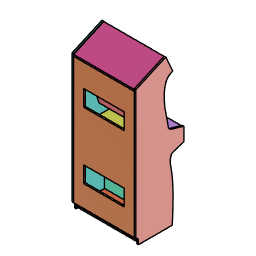
arcade_design (Autodesk Fusion 360 design; units mm, degrees)
Autodesk Fusion 360 part; units mm, degrees
sketch "Side Panels" plane through (0, 0, 0) normal (1, 0, 0) x (0, 1, 0)
  line L0 (31.75, 0) -> (457.2, 0)
  line L1 (452.7885, 785.6533) -> (609.6, 837.3077)
  line L2 (609.6, 837.3077) -> (609.6, 1002.4077)
  line L3 (609.6, 1002.4077) -> (444.4309, 1049.7691)
  line L4 (408.5002, 1089.2565) -> (363.7179, 1328.5488)
  line L5 (463.7201, 1671.9295) -> (375.9057, 1869.164)
  line L6 (0, 82.55) -> (0, 1701.8)
  line L7 (375.9057, 1869.164) -> (0, 1701.8)
  line L8 (0, 0) -> (31.75, 0)
  line L9 (31.75, 0) -> (31.75, 50.8)
  arc A0 (31.75, 50.8) -> (0, 82.55) centre (0, 50.8) ccw
  spline S0 degree 5 poles (463.7201, 1671.9295) (458.0026, 1670.3002) (446.9286, 1666.533) (431.4003, 1659.3565) (412.8977, 1646.6853) (393.6414, 1625.3901) (378.472, 1598.336) (367.4495, 1565.4385) (360.3055, 1527.0756) (356.6509, 1483.7958) (356.0894, 1436.1574) (357.8593, 1394.9197) (360.3453, 1362.3589) (362.5093, 1339.9378) (363.7179, 1328.5488) knots 0 0 0 0 0 0 0.1 0.2 0.3 0.4 0.5 0.6 0.7 0.8 0.9 1 1 1 1 1 1
  spline S1 degree 5 poles (452.7885, 785.6533) (450.1173, 780.6819) (445.2009, 770.7662) (439.1046, 755.9734) (433.5518, 736.4131) (430.8508, 711.9873) (432.0376, 686.8334) (436.2286, 659.4045) (442.2622, 627.782) (448.9298, 590.0685) (455.2454, 544.8887) (460.5567, 491.5686) (464.4393, 429.8652) (466.6536, 359.8453) (467.0872, 281.7419) (465.7134, 195.857) (463.1837, 121.152) (460.4968, 61.8426) (458.357, 20.8555) (457.2, 0) knots 0 0 0 0 0 0 0.066667 0.133333 0.2 0.266667 0.333333 0.4 0.466667 0.533333 0.6 0.666667 0.733333 0.8 0.866667 0.933333 1 1 1 1 1 1
  arc A1 (408.5002, 1089.2565) -> (444.4309, 1049.7691) centre (458.4333, 1098.6012) ccw
  point P0 (414.2716, 1058.4172)
  point P1 (31.75, 82.55)
  point P2 (381, 1600.2)
  point P3 (431.8, 711.2)
  point P4 (446.1027, 605.186)
  dimension "d1" = 457.2
  dimension "d3" = 165.1
  dimension "d5" = 165.1
  dimension "d6" = 203.2
  dimension "d7" = 106
  dimension "d8" = 10.6
  dimension "d9" = 1701.8
  dimension "d10" = 411.48
  dimension "d11" = 114
  dimension "d12" = 215.9
  dimension "d13" = 31.75
  dimension "d14" = 82.55
  dimension "d15" = 31.75
  dimension "d18" = 50.8
  dimension "d37" = 609.6
  constraint coincident L8.start origin
  constraint horizontal L0
  constraint vertical L2
  constraint perpendicular L0 L6
  constraint coincident L6 L7.end
  constraint perpendicular L5 L7
  constraint perpendicular L6 L8
  constraint perpendicular L0 L9
  constraint coincident P1 L9
  constraint tangent L9 A0
  constraint coincident P0 L3
  constraint coincident P0 L4
  constraint tangent L3 A1
  constraint tangent L4 A1
  measures "d1" distance of L8.start L0.end
  measures "d3" distance of L1.start L1.end
  measures "d5" distance of L1.end L2.end
  measures "d6" distance of L2.end P0
  measures "d7" angle of L2 L3
  measures "d8" angle of L4 L6
  measures "d9" distance of L8.start L6.end
  measures "d10" distance of L5.end L6.end
  measures "d11" angle of L6 L7
  measures "d12" distance of L5.start L5.end
  measures "d13" distance of L8.start L0.start
  measures "d14" distance of L0.start P1
  measures "d15" radius of A0
  measures "d18" radius of A1
  measures "d37" distance of L2 L6
extrude "Extrude1" add sketch "Side Panels" along normal blind 19.05 makes body 1 in component "Right Panel"
extrude "Extrude1'" add sketch "Side Panels" along normal blind 19.05 separate body makes body 2 in component "Left Panel"
sketch "Main Panels" plane through (19.05, 0, 0) normal (1, 0, 0) x (0, 1, 0)
  line L0 (463.7201, 1671.9295) -> (375.9057, 1869.164)
  line L1 (375.9057, 1869.164) -> (0, 1701.8)
  line L2 (0, 1701.8) -> (0, 82.55)
  arc A0 (31.75, 50.8) -> (0, 82.55) centre (0, 50.8) ccw
  line L3 (31.75, 50.8) -> (31.75, 0)
  line L4 (31.75, 0) -> (457.2, 0)
  spline S0 degree 5 poles (457.2, 0) (458.357, 20.8555) (460.4968, 61.8426) (463.1837, 121.152) (465.7134, 195.857) (467.0872, 281.7419) (466.6536, 359.8453) (464.4393, 429.8652) (460.5567, 491.5686) (455.2454, 544.8887) (448.9298, 590.0685) (442.2622, 627.782) (436.2286, 659.4045) (432.0376, 686.8334) (430.8508, 711.9873) (433.5518, 736.4131) (439.1046, 755.9734) (445.2009, 770.7662) (450.1173, 780.6819) (452.7885, 785.6533) knots -1 -1 -1 -1 -1 -1 -0.933333 -0.866667 -0.8 -0.733333 -0.666667 -0.6 -0.533333 -0.466667 -0.4 -0.333333 -0.266667 -0.2 -0.133333 -0.066667 0 0 0 0 0 0
  line L5 (452.7885, 785.6533) -> (609.6, 837.3077)
  line L6 (609.6, 837.3077) -> (609.6, 1002.4077)
  line L7 (609.6, 1002.4077) -> (444.4309, 1049.7691)
  arc A1 (408.5002, 1089.2565) -> (444.4309, 1049.7691) centre (458.4333, 1098.6012) ccw
  line L8 (408.5002, 1089.2565) -> (363.7179, 1328.5488)
  spline S1 degree 5 poles (363.7179, 1328.5488) (362.5093, 1339.9378) (360.3453, 1362.3589) (357.8593, 1394.9197) (356.0894, 1436.1574) (356.6509, 1483.7958) (360.3055, 1527.0756) (367.4495, 1565.4385) (378.472, 1598.336) (393.6414, 1625.3901) (412.8977, 1646.6853) (431.4003, 1659.3565) (446.9286, 1666.533) (458.0026, 1670.3002) (463.7201, 1671.9295) knots -1 -1 -1 -1 -1 -1 -0.9 -0.8 -0.7 -0.6 -0.5 -0.4 -0.3 -0.2 -0.1 0 0 0 0 0 0
  line L9 (375.9057, 1869.164) -> (383.654, 1851.761)
  line L10 (383.654, 1851.761) -> (0, 1680.9472)
  line L11 (0, 1680.9472) -> (0, 1701.8)
  line L12 (0, 1701.8) -> (375.9057, 1869.164)
  line L13 (0, 1680.9472) -> (0, 82.55)
  line L14 (0, 82.55) -> (19.05, 82.55)
  line L15 (19.05, 82.55) -> (19.05, 1689.4288)
  line L16 (463.7201, 1671.9295) -> (455.9718, 1689.3326)
  line L17 (455.9718, 1689.3326) -> (160.5069, 1557.7831)
  line L18 (166.4261, 1539.5657) -> (463.7201, 1671.9295)
  line L19 (406.3216, 0) -> (406.3216, 862.4074)
  line L20 (406.3216, 862.4074) -> (387.2716, 862.4074)
  line L21 (387.2716, 862.4074) -> (387.2716, 0)
  line L22 (565.0941, 983.0574) -> (584.1441, 983.0574)
  line L23 (584.1441, 983.0574) -> (584.1441, 881.4574)
  line L24 (584.1441, 881.4574) -> (565.0941, 881.4574)
  line L25 (565.0941, 881.4574) -> (565.0941, 983.0574)
  line L26 (565.0941, 881.4574) -> (565.0941, 862.4074)
  line L27 (565.0941, 862.4074) -> (184.0941, 862.4074)
  line L28 (184.0941, 862.4074) -> (184.0941, 881.4574)
  line L29 (184.0941, 881.4574) -> (565.0941, 881.4574)
  line L30 (598.8774, 1003.0679) -> (597.2171, 984.0904)
  line L31 (597.2171, 984.0904) -> (339.5874, 1006.63)
  line L32 (333.1923, 1026.3123) -> (598.8774, 1003.0679)
  line L33 (565.0941, 983.0574) -> (355.6, 983.0574) construction
  line L34 (333.1923, 1026.3123) -> (166.4261, 1539.5657)
  line L35 (333.1923, 1026.3123) -> (339.5874, 1006.63)
  line L36 (166.4261, 1539.5657) -> (160.5069, 1557.7831)
  line L37 (154.343, 1576.7538) -> (136.2254, 1570.867)
  line L38 (136.2254, 1570.867) -> (321.4698, 1000.7433)
  line L39 (339.5874, 1006.63) -> (321.4698, 1000.7433)
  line L40 (154.343, 1576.7538) -> (166.4261, 1539.5657)
  dimension "d19" = 19.05
  dimension "d20" = 19.05
  dimension "d21" = 19.05
  dimension "d23" = 19.05
  dimension "d27" = 19.05
  dimension "d28" = 101.6
  dimension "d29" = 19.05
  dimension "d30" = 381
  dimension "d31" = 19.05
  dimension "d32" = 266.7
  dimension "d33" = 5
  dimension "d34" = 18
  dimension "d36" = 19.05
  constraint coincident L0.end L1.start
  constraint coincident L0 L9.end
  constraint coincident L2 L10.end
  constraint perpendicular L0 L10
  constraint coincident L1.end L2.start
  constraint coincident L2.end A0.end
  constraint perpendicular L2 L14
  constraint coincident L10 L15.end
  constraint perpendicular L14 L15
  constraint coincident L0.start S1.end
  constraint parallel L0 L16
  constraint perpendicular L0 L17
  constraint perpendicular L0 L18
  constraint coincident L4 L19.start
  constraint perpendicular L4 L19
  constraint perpendicular L19 L20
  constraint coincident L4 L21.end
  constraint perpendicular L4 L21
  constraint horizontal L22
  constraint perpendicular L22 L23
  constraint perpendicular L23 L24
  constraint perpendicular L22 L25
  constraint perpendicular L24 L26
  constraint perpendicular L21 L27
  constraint perpendicular L27 L28
  constraint perpendicular L30 L31
  constraint parallel L31 L32
  constraint perpendicular L25 L33
  constraint coincident L19.end L27
  constraint parallel L34 L35
  constraint parallel L34 L36
  constraint perpendicular L36 L37
  constraint perpendicular L37 L38
  constraint perpendicular L38 L39
  constraint perpendicular L37 L40
  measures "d19" distance of L0.end L9.end
  measures "d20" distance of L2.end L14.end
  measures "d21" distance of L0.start L16.end
  measures "d23" distance of L19.end L20.end
  measures "d27" distance of L22.start L22.end
  measures "d28" distance of L22.end L23.end
  measures "d29" distance of L24.end L26.end
  measures "d30" distance of L26.end L27.end
  measures "d31" distance of L30.start L30.end
  measures "d32" distance of L30.start L32.start
  measures "d33" angle of L31 L33
  measures "d34" angle of L15 L34
  measures "d36" distance of L37.start L37.end
extrude "Extrude1''" add sketch "Main Panels" along normal blind 711.2 separate body contours L2 L10 L13 L14 L15 makes body 3 in component "Back Panel"
extrude "Extrude1'''" add sketch "Main Panels" along normal blind 711.2 separate body contours L34 L35 L36 L37 L38 L39 L40 makes body 4 in component "Screen Panel"
extrude "Extrude1''''" add sketch "Main Panels" along normal blind 711.2 separate body contours L30 L31 L32 L35 makes body 5 in component "Control Panel"
extrude "Extrude1'''''" add sketch "Main Panels" along normal blind 711.2 separate body contours L22 L23 L24 L25 makes body 6 in component "Tray Door"
extrude "Extrude1''''''" add sketch "Main Panels" along normal blind 711.2 separate body contours L20 L26 L27 L28 L29 makes body 7 in component "Tray Bottom"
extrude "Extrude1'''''''" add sketch "Main Panels" along normal blind 711.2 separate body contours L4 L19 L20 L21 L27 makes body 8 in component "Front Panel"
sketch "Keyboard Tray" plane through (19.05, 0, 0) normal (1, 0, 0) x (0, 1, 0)
  line L0 (463.7201, 1671.9295) -> (375.9057, 1869.164)
  line L1 (375.9057, 1869.164) -> (0, 1701.8)
  line L2 (0, 1701.8) -> (0, 82.55)
  arc A0 (31.75, 50.8) -> (0, 82.55) centre (0, 50.8) ccw
  line L3 (31.75, 50.8) -> (31.75, 0)
  line L4 (31.75, 0) -> (457.2, 0)
  spline S0 degree 5 poles (457.2, 0) (458.357, 20.8555) (460.4968, 61.8426) (463.1837, 121.152) (465.7134, 195.857) (467.0872, 281.7419) (466.6536, 359.8453) (464.4393, 429.8652) (460.5567, 491.5686) (455.2454, 544.8887) (448.9298, 590.0685) (442.2622, 627.782) (436.2286, 659.4045) (432.0376, 686.8334) (430.8508, 711.9873) (433.5518, 736.4131) (439.1046, 755.9734) (445.2009, 770.7662) (450.1173, 780.6819) (452.7885, 785.6533) knots -1 -1 -1 -1 -1 -1 -0.933333 -0.866667 -0.8 -0.733333 -0.666667 -0.6 -0.533333 -0.466667 -0.4 -0.333333 -0.266667 -0.2 -0.133333 -0.066667 0 0 0 0 0 0
  line L5 (452.7885, 785.6533) -> (609.6, 837.3077)
  line L6 (609.6, 837.3077) -> (609.6, 1002.4077)
  line L7 (609.6, 1002.4077) -> (444.4309, 1049.7691)
  arc A1 (408.5002, 1089.2565) -> (444.4309, 1049.7691) centre (458.4333, 1098.6012) ccw
  line L8 (408.5002, 1089.2565) -> (363.7179, 1328.5488)
  spline S1 degree 5 poles (363.7179, 1328.5488) (362.5093, 1339.9378) (360.3453, 1362.3589) (357.8593, 1394.9197) (356.0894, 1436.1574) (356.6509, 1483.7958) (360.3055, 1527.0756) (367.4495, 1565.4385) (378.472, 1598.336) (393.6414, 1625.3901) (412.8977, 1646.6853) (431.4003, 1659.3565) (446.9286, 1666.533) (458.0026, 1670.3002) (463.7201, 1671.9295) knots -1 -1 -1 -1 -1 -1 -0.9 -0.8 -0.7 -0.6 -0.5 -0.4 -0.3 -0.2 -0.1 0 0 0 0 0 0
  line L9 (267.3124, 912.0538) -> (546.7124, 912.0538)
  line L10 (546.7124, 912.0538) -> (546.7124, 893.0038)
  line L11 (546.7124, 893.0038) -> (267.3124, 893.0038)
  line L12 (267.3124, 893.0038) -> (267.3124, 912.0538)
  dimension "d54" = 279.4
  dimension "d55" = 19.05
  constraint horizontal L9
  constraint vertical L10
  constraint horizontal L11
  constraint vertical L12
  measures "d54" distance of L9.start L9.end
  measures "d55" distance of L9.start L11.end
extrude "Extrude1''''''''" add sketch "Keyboard Tray" along normal blind 711.2 separate body contours L9 L10 L11 L12 makes body 9 in component "Keyboard Tray"
sketch "Coin Door" plane through (0, 406.3216, 0) normal (0, 1, 0) x (-1, 0, 0)
  line L0 (-19.05, 0) -> (-19.05, 862.4074)
  line L1 (-19.05, 862.4074) -> (-730.25, 862.4074)
  line L2 (-730.25, 862.4074) -> (-730.25, 0)
  line L3 (-730.25, 0) -> (-19.05, 0)
  line L4 (-730.25, 509.3131) -> (-19.05, 509.3131) construction
  line L5 (-287.02, 633.7731) -> (-462.28, 633.7731)
  line L6 (-462.28, 633.7731) -> (-462.28, 384.8531)
  line L7 (-462.28, 384.8531) -> (-287.02, 384.8531)
  line L8 (-287.02, 384.8531) -> (-287.02, 633.7731)
  line L9 (-287.02, 633.7731) -> (-462.28, 384.8531) construction
  line L10 (-462.28, 633.7731) -> (-287.02, 384.8531) construction
  point P0 (-374.65, 509.3131)
  dimension "d70" = 175.26
  dimension "d71" = 248.92
  constraint horizontal L4
  constraint coincident L2 L4.start
  constraint coincident L0 L4.end
  constraint horizontal L5
  constraint perpendicular L5 L6
  constraint parallel L5 L7
  constraint parallel L6 L8
  constraint coincident L9 P0
  constraint coincident L10 P0
  constraint midpoint L4 P0
  measures "d70" distance of L6.end L7.end
  measures "d71" distance of L5.end L6.end
extrude "Extrude2" cut sketch "Coin Door" against normal blind 25.4 contours L5 L6 L7 L8 bodies 8 in component "Front Panel"
sketch "Sketch5" plane through (781.05, 0, 0) normal (-1, 0, 0) x (0, -1, 0)
  line L0 (-375.9057, 1869.164) -> (-463.7201, 1671.9295)
  spline S0 degree 5 poles (-463.7201, 1671.9295) (-458.0026, 1670.3002) (-446.9286, 1666.533) (-431.4003, 1659.3565) (-412.8977, 1646.6853) (-393.6414, 1625.3901) (-378.472, 1598.336) (-367.4495, 1565.4385) (-360.3055, 1527.0756) (-356.6509, 1483.7958) (-356.0894, 1436.1574) (-357.8593, 1394.9197) (-360.3453, 1362.3589) (-362.5093, 1339.9378) (-363.7179, 1328.5488) knots 0 0 0 0 0 0 0.1 0.2 0.3 0.4 0.5 0.6 0.7 0.8 0.9 1 1 1 1 1 1
  line L1 (-363.7179, 1328.5488) -> (-408.5002, 1089.2565)
  arc A0 (-444.4309, 1049.7691) -> (-408.5002, 1089.2565) centre (-458.4333, 1098.6012) ccw
  line L2 (-444.4309, 1049.7691) -> (-609.6, 1002.4077)
  line L3 (-609.6, 1002.4077) -> (-609.6, 837.3077)
  line L4 (-609.6, 837.3077) -> (-452.7885, 785.6533)
  spline S1 degree 5 poles (-452.7885, 785.6533) (-450.1173, 780.6819) (-445.2009, 770.7662) (-439.1046, 755.9734) (-433.5518, 736.4131) (-430.8508, 711.9873) (-432.0376, 686.8334) (-436.2286, 659.4045) (-442.2622, 627.782) (-448.9298, 590.0685) (-455.2454, 544.8887) (-460.5567, 491.5686) (-464.4393, 429.8652) (-466.6536, 359.8453) (-467.0872, 281.7419) (-465.7134, 195.857) (-463.1837, 121.152) (-460.4968, 61.8426) (-458.357, 20.8555) (-457.2, 0) knots 0 0 0 0 0 0 0.066667 0.133333 0.2 0.266667 0.333333 0.4 0.466667 0.533333 0.6 0.666667 0.733333 0.8 0.866667 0.933333 1 1 1 1 1 1
  line L5 (-457.2, 0) -> (-31.75, 0)
  line L6 (-31.75, 0) -> (-31.75, 50.8)
  arc A1 (0, 82.55) -> (-31.75, 50.8) centre (0, 50.8) ccw
  line L7 (0, 82.55) -> (0, 1701.8)
  line L8 (0, 1701.8) -> (-375.9057, 1869.164)
  line L9 (-387.2716, 25.3658) -> (-31.75, 25.3658)
  line L10 (-31.75, 25.3658) -> (-31.75, 44.4158)
  line L11 (-31.75, 44.4158) -> (-387.2716, 44.4158)
  line L12 (-387.2716, 44.4158) -> (-387.2716, 25.3658)
  line L13 (-387.2716, 862.4074) -> (-387.2716, 0)
  dimension "d74" = 19.05
  constraint horizontal L9
  constraint vertical L10
  constraint horizontal L11
  constraint vertical L12
  constraint coincident L6 L10.end
  constraint coincident L9.start L13
  measures "d74" distance of L9.start L11.end
extrude "Extrude1'''''''''" add sketch "Sketch5" along normal blind 711.2 separate body contours L6 L9 L10 L11 L12 L13 makes body 10 in component "Bottom Panel"
sketch "Access" plane through (0, 0, 0) normal (0, -1, 0) x (1, 0, 0) in component "Back Panel"
  line L0 (19.05, 1680.9472) -> (19.05, 82.55)
  line L1 (19.05, 82.55) -> (730.25, 82.55)
  line L2 (730.25, 82.55) -> (730.25, 1680.9472)
  line L3 (730.25, 1680.9472) -> (19.05, 1680.9472)
  line L4 (19.05, 1570.867) -> (19.05, 1000.7433) construction
  line L5 (19.05, 1285.8052) -> (730.25, 1285.8052) construction
  line L6 (19.05, 455.2789) -> (730.25, 455.2789) construction
  line L7 (628.65, 1387.4052) -> (120.65, 1387.4052)
  line L8 (120.65, 1387.4052) -> (120.65, 1184.2052)
  line L9 (120.65, 1184.2052) -> (628.65, 1184.2052)
  line L10 (628.65, 1184.2052) -> (628.65, 1387.4052)
  line L11 (628.65, 1387.4052) -> (120.65, 1184.2052) construction
  line L12 (120.65, 1387.4052) -> (628.65, 1184.2052) construction
  line L13 (628.65, 556.8789) -> (120.65, 556.8789)
  line L14 (120.65, 556.8789) -> (120.65, 353.6789)
  line L15 (120.65, 353.6789) -> (628.65, 353.6789)
  line L16 (628.65, 353.6789) -> (628.65, 556.8789)
  line L17 (628.65, 556.8789) -> (120.65, 353.6789) construction
  line L18 (120.65, 556.8789) -> (628.65, 353.6789) construction
  point P0 (374.65, 1285.8052)
  point P1 (374.65, 455.2789)
  dimension "d77" = 508
  dimension "d78" = 203.2
  dimension "d79" = 508
  dimension "d80" = 203.2
  constraint horizontal L5
  constraint midpoint L4 L5.start
  constraint coincident L2 L5.end
  constraint coincident L0 L6.start
  constraint coincident L2 L6.end
  constraint perpendicular L2 L6
  constraint horizontal L7
  constraint perpendicular L7 L8
  constraint parallel L7 L9
  constraint parallel L8 L10
  constraint coincident L11 P0
  constraint coincident L12 P0
  constraint midpoint L5 P0
  constraint horizontal L13
  constraint perpendicular L13 L14
  constraint parallel L13 L15
  constraint parallel L14 L16
  constraint coincident L17 P1
  constraint coincident L18 P1
  constraint midpoint L6 P1
  measures "d77" distance of L8.end L9.end
  measures "d78" distance of L7.end L8.end
  measures "d79" distance of L14.end L15.end
  measures "d80" distance of L13.end L14.end
extrude "Extrude2'" cut sketch "Access" against normal blind 25.4 contours L7 L8 L9 L10 bodies 3 in component "Back Panel"
extrude "Extrude3" cut sketch "Access" against normal blind 25.4 contours L13 L14 L15 L16 bodies 3 in component "Back Panel"
sketch "Sketch1" plane through (19.05, 0, 0) normal (-1, 0, 0) x (0, -1, 0) in component "Screen Panel"
  line L0 (-321.4698, 1000.7433) -> (-136.2254, 1570.867)
  line L1 (-136.2254, 1570.867) -> (-154.343, 1576.7538)
  line L2 (-154.343, 1576.7538) -> (-339.5874, 1006.63)
  line L3 (-339.5874, 1006.63) -> (-321.4698, 1000.7433)
  line L4 (-339.5874, 1006.63) -> (-597.2171, 984.0904)
  line L5 (-318.971, 1008.4337) -> (-321.4698, 1000.7433)
  line L6 (-339.5874, 1006.63) -> (-318.971, 1008.4337)
  constraint coincident L0 L5.start
  constraint coincident L0.start L3.end
  constraint perpendicular L3 L5
  constraint coincident L2.end L3.start
  constraint parallel L4 L6
extrude "Extrude2''" cut sketch "Sketch1" against normal blind 711.2 contours L0 L3 L5 L6 bodies 4 in component "Screen Panel"
move_face "OffsetFaces1" offset -6.35 1 faces at (256.1167, 12.7, 1686.6016) on bodies 3 in component "Back Panel"
sketch "Sketch6" plane through (781.05, 0, 0) normal (-1, 0, 0) x (0, -1, 0)
  line L0 (0, 82.55) -> (0, 1701.8)
  line L1 (0, 1673.9962) -> (0, 1694.8491)
  line L2 (-463.7201, 1671.9295) -> (-375.9057, 1869.164)
  line L3 (0, 1694.8491) -> (-378.4885, 1863.363)
  line L4 (0, 1673.9962) -> (-386.2368, 1845.9599)
  line L5 (-386.2368, 1845.9599) -> (-378.4885, 1863.363)
  line L6 (-339.5874, 1006.63) -> (-154.343, 1576.7538)
  line L7 (-461.1373, 1677.7305) -> (-164.4531, 1545.6382)
  line L8 (-461.1373, 1677.7305) -> (-453.389, 1695.1336)
  line L9 (-453.389, 1695.1336) -> (-158.5339, 1563.8556)
  line L10 (-158.5339, 1563.8556) -> (-164.4531, 1545.6382)
  point P0 (0, 1673.9962)
  dimension "d88" = 19.05
  dimension "d89" = 6.35
  dimension "d90" = 19.05
  dimension "d91" = 6.35
  constraint coincident P0 L1.start
  constraint coincident L0 L1.end
  constraint parallel L0 L1
  constraint coincident L2 L3.end
  constraint perpendicular L2 L3
  constraint coincident L2 L4.end
  constraint perpendicular L2 L4
  constraint coincident L2 L7.start
  constraint coincident L6 L7.end
  constraint perpendicular L2 L7
  constraint perpendicular L7 L8
  constraint coincident L6 L9.end
  constraint perpendicular L2 L9
  measures "d88" distance of L3 L4
  measures "d89" distance of L2.end L3.end
  measures "d90" distance of L7.start L8.end
  measures "d91" distance of L2.start L7.start
extrude "Extrude1''''''''''" add sketch "Sketch6" along normal blind 711.2 separate body contours L2 L6 L7 L8 L9 L10 makes body 11 in component "Marquee Bottom"
extrude "Extrude1'''''''''''" add sketch "Sketch6" along normal blind 711.2 separate body contours L0 L1 L2 L3 L4 L5 makes body 12 in component "Marquee Top"
move_face "OffsetFaces1'" offset -6.35 1 faces at (6.35, 609.6, 892.341) on bodies 1 in component "Right Panel"
move_face "OffsetFaces1''" offset -6.35 1 faces at (6.35, 609.6, 892.341) on bodies 2 in component "Left Panel"
move_face "OffsetFaces1'''" offset -6.35 1 faces at (256.1167, 598.324, 996.742) on bodies 5 in component "Control Panel"
move_body "Move1" bodies 6 to x (1, 0, 0) y (0, 1, 0) z (0, 0, 1) at (0, -6.35, 0) in component "Tray Door"
move_body "Move1'" bodies 7 to x (1, 0, 0) y (0, 1, 0) z (0, 0, 1) at (0, -6.35, 0) in component "Tray Bottom"
extrude "Extrude3'" cut 1 faces at (256.1167, 399.9716, 862.4074) along direction (0, 0, -1) blind 33.02 on bodies 8 bodies 8 in component "Front Panel"
move_body "Move1''" bodies 9 to x (1, 0, 0) y (0, 1, 0) z (0, 0, 1) at (0, 0, -33.02) in component "Keyboard Tray"
move_body "Move2" bodies 7 to x (1, 0, 0) y (0, 1, 0) z (0, 0, 1) at (0, 0, -33.02) in component "Tray Bottom"
extrude "Extrude2'''" add 1 faces at (256.1167, 571.4441, 881.4574) along direction (0, 0, -1) blind 33.02 on bodies 6 bodies 6 in component "Tray Door"
extrude "Extrude3''" add 1 faces at (730.25, 270.9671, 1197.2725) along direction (1, 0, 0) blind 50.8 on bodies 4 bodies 4 in component "Screen Panel"
extrude "Extrude2''''" add 1 faces at (730.25, 421.7771, 1012.1879) along direction (1, 0, 0) blind 50.8 on bodies 5 bodies 5 in component "Control Panel"
extrude "Extrude3'''" add 1 faces at (730.25, 565.0941, 893.3107) along direction (1, 0, 0) blind 50.8 on bodies 6 bodies 6 in component "Tray Door"
extrude "Extrude2'''''" add 1 faces at (730.25, 360.4457, 872.6838) along direction (1, 0, 0) blind 50.8 on bodies 9 bodies 9 in component "Keyboard Tray"
extrude "Extrude2''''''" add 1 faces at (730.25, 378.8199, 842.0874) along direction (1, 0, 0) blind 50.8 on bodies 7 bodies 7 in component "Tray Bottom"
extrude "Extrude4" add 1 faces at (730.25, 393.6216, 552.9249) along direction (1, 0, 0) blind 50.8 on bodies 8 bodies 8 in component "Front Panel"
extrude "Extrude4'" add 1 faces at (730.25, 12.7, 1146.3414) along direction (1, 0, 0) blind 50.8 on bodies 3 bodies 3 in component "Back Panel"
extrude "Extrude2'''''''" add 1 faces at (69.85, 128.7456, 1738.2684) along direction (-1, 0, 0) blind 50.8 on bodies 12 bodies 12 in component "Marquee Top"
extrude "Extrude2''''''''" add 1 faces at (69.85, 261.3748, 1595.7414) along direction (-1, 0, 0) blind 50.8 on bodies 11 bodies 11 in component "Marquee Bottom"
extrude "Extrude2'''''''''" add 1 faces at (69.85, 150.2572, 31.7158) along direction (-1, 0, 0) blind 50.8 on bodies 10 bodies 10 in component "Bottom Panel"
extrude "Extrude5" add 1 faces at (287.02, 393.6216, 550.7997) along direction (1, 0, 0) blind 25.4 on bodies 8 bodies 8 in component "Front Panel"
extrude "Extrude6" cut 1 faces at (462.28, 393.6216, 550.7997) along direction (1, 0, 0) blind 25.4 on bodies 8 bodies 8 in component "Front Panel"
extrude "Extrude5'" add 1 faces at (120.65, 6.35, 421.4123) along direction (1, 0, 0) blind 25.4 on bodies 3 bodies 3 in component "Back Panel"
extrude "Extrude6'" cut 1 faces at (628.65, 6.35, 421.4123) along direction (1, 0, 0) blind 25.4 on bodies 3 bodies 3 in component "Back Panel"
extrude "Extrude7" add 1 faces at (120.65, 12.7, 1251.9385) along direction (1, 0, 0) blind 25.4 on bodies 3 bodies 3 in component "Back Panel"
extrude "Extrude8" cut 1 faces at (628.65, 6.35, 1251.9385) along direction (1, 0, 0) blind 25.4 on bodies 3 bodies 3 in component "Back Panel"
extrude "Extrude4''" add 1 faces at (527.05, 142.2646, 1572.8293) along direction (0, -0.309017, 0.951057) blind 50.8 on bodies 4 bodies 4 in component "Screen Panel"
component "Right Panel" placed x (1, 0, 0) y (0, 1, 0) z (0, 0, 1) at (0, 0, 0)
component "Left Panel" placed x (1, 0, 0) y (0, 1, 0) z (0, 0, 1) at (781.05, 0, 0)
component "Back Panel" placed x (1, 0, 0) y (0, 1, 0) z (0, 0, 1) at (0, 0, 0)
component "Screen Panel" placed x (1, 0, 0) y (0, 1, 0) z (0, 0, 1) at (0, 0, 0)
component "Control Panel" placed x (1, 0, 0) y (0, 1, 0) z (0, 0, 1) at (0, 0, 0)
component "Tray Door" placed x (1, 0, 0) y (0, 1, 0) z (0, 0, 1) at (0, 0, 0)
component "Tray Bottom" placed x (1, 0, 0) y (0, 1, 0) z (0, 0, 1) at (0, 0, 0)
component "Front Panel" placed x (1, 0, 0) y (0, 1, 0) z (0, 0, 1) at (0, 0, 0)
component "Keyboard Tray" placed x (1, 0, 0) y (0, 1, 0) z (0, 0, 1) at (0, 0, 0)
component "Bottom Panel" placed x (1, 0, 0) y (0, 1, 0) z (0, 0, 1) at (0, 0, 0)
component "Marquee Bottom" placed x (1, 0, 0) y (0, 1, 0) z (0, 0, 1) at (0, 0, 0)
component "Marquee Top" placed x (1, 0, 0) y (0, 1, 0) z (0, 0, 1) at (0, 0, 0)
equation "BoardThickness = ( 3 / 4 ) * 1 in"
equation "BoardThickness_1 = ( 3 / 4 ) * 1 in"
equation "d19 = BoardThickness"
equation "d20 = BoardThickness"
equation "d21 = BoardThickness"
equation "d23 = BoardThickness"
equation "d27 = BoardThickness"
equation "d29 = BoardThickness"
equation "d31 = BoardThickness"
equation "d36 = BoardThickness"
equation "d55 = BoardThickness"
equation "d74 = BoardThickness"
equation "d88 = BoardThickness"
equation "d90 = BoardThickness"
named bodies: "Right Panel", "Left Panel", "Back Panel", "Screen Panel", "Control Panel", "Tray Door", "Tray Bottom", "Front Panel", "Keyboard Tray", "Bottom Panel", "Marquee Bottom", "Marquee Top"
